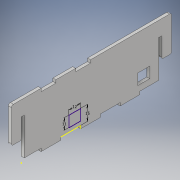
# Autodesk Inventor part: side_v2
Saved by Autodesk Inventor 2017.2 (Build 212233000, 233)
## iProperties
Created: 2017-06-09
Part Number: side_v2
Material: Generic
Document SubType Name: Modeling
Designer: SandeepSH
Density: 1 g/cm^3
Appearance: Default
Author: SandeepSH
Autodesk Inventor part; units mm, degrees
ref_plane "YZ Plane" through (0, 0, 0) normal (1, 0, 0) x (0, 1, 0)
ref_plane "XZ Plane" through (0, 0, 0) normal (0, 1, 0) x (-1, 0, 0)
ref_plane "XY Plane" through (0, 0, 0) normal (0, 0, 1) x (1, 0, 0)
sketch "Sketch1" plane through (0, 0, 0) normal (1, 0, 0) x (0, 1, 0)
  line L0 (0, 0) -> (55.5, 0)
  line L1 (55.5, 0) -> (55.5, -142)
  line L2 (55.5, -142) -> (0, -142)
  line L3 (0, -142) -> (0, 0)
  dimension "d0" = 55.5
  dimension "d1" = 142
  constraints: 8 end point, 2 parallel, 1 horizontal, 1 perpendicular
  measures "d0" distance of L1.end L2.end
  measures "d1" distance of L0.end L1.end
extrude "Extrusion1" add sketch "Sketch1" along normal blind 3
sketch "Sketch2" plane through (3, 0, 0) normal (1, 0, 0) x (0, 0, -1)
  line L0 (0, 0) -> (142, 0) projected
  line L1 (0, 0) -> (20, 0)
  line L2 (20, 0) -> (20, 3)
  line L3 (20, 3) -> (0, 3)
  line L4 (0, 3) -> (0, 0)
  line L5 (40, 0) -> (60, 0)
  line L6 (60, 0) -> (60, 3)
  line L7 (60, 3) -> (40, 3)
  line L8 (40, 3) -> (40, 0)
  line L9 (80, 0) -> (100, 0)
  line L10 (100, 0) -> (100, 3)
  line L11 (100, 3) -> (80, 3)
  line L12 (80, 3) -> (80, 0)
  line L13 (142, 0) -> (120, 0)
  line L14 (120, 0) -> (120, 3)
  line L15 (120, 3) -> (142, 3)
  line L16 (142, 3) -> (142, 0)
  line L17 (142, 55.5) -> (0, 55.5) projected
  line L18 (20, 55.5) -> (35, 55.5)
  line L19 (35, 55.5) -> (35, 52.5)
  line L20 (35, 52.5) -> (20, 52.5)
  line L21 (20, 52.5) -> (20, 55.5)
  line L22 (0, 55.5) -> (0, 0) projected
  line L23 (55, 55.5) -> (70, 55.5)
  line L24 (70, 55.5) -> (70, 52.5)
  line L25 (70, 52.5) -> (55, 52.5)
  line L26 (55, 52.5) -> (55, 55.5)
  line L27 (0, 3) -> (3, 3)
  line L28 (3, 3) -> (3, 40.5)
  line L29 (3, 40.5) -> (0, 40.5)
  line L30 (0, 40.5) -> (0, 3)
  line L31 (142, 3) -> (139, 3)
  line L32 (139, 3) -> (139, 40.5)
  line L33 (139, 40.5) -> (142, 40.5)
  line L34 (142, 40.5) -> (142, 3)
  dimension "d4" = 20
  dimension "d5" = 3
  dimension "d6" = 20
  dimension "d7" = 20
  dimension "d8" = 3
  dimension "d9" = 20
  dimension "d10" = 20
  dimension "d11" = 3
  dimension "d12" = 20
  dimension "d13" = 15
  dimension "d14" = 3
  dimension "d17" = 20
  dimension "d18" = 15
  dimension "d19" = 20
  dimension "d20" = 3
  dimension "d21" = 15
  dimension "d22" = 3
  dimension "d23" = 15
  constraints: 64 end point, 16 parallel, 8 horizontal, 8 perpendicular, 5 point on line
  measures "d4" distance of L3.end L2.end
  measures "d5" distance of L2.end L1.end
  measures "d6" distance of L7.end L6.end
  measures "d7" distance of L11.end L10.end
  measures "d8" distance of L10.end L9.end
  measures "d9" distance between parallel lines of L8 L2
  measures "d10" distance between parallel lines of L12 L6
  measures "d11" distance of L13.end L14.end
  measures "d12" distance between parallel lines of L14 L10
  measures "d13" distance of L19.end L20.end
  measures "d14" distance of L18.end L19.end
  measures "d17" distance between parallel lines of L21 L22
  measures "d18" distance of L24.end L25.end
  measures "d19" distance between parallel lines of L26 L19
  measures "d20" distance of L29.end L28.end
  measures "d21" distance between parallel lines of L17 L29
  measures "d22" distance of L32.end L33.end
  measures "d23" distance between parallel lines of L17 L33
extrude "Extrusion2" cut sketch "Sketch2" against normal through all
sketch "Sketch3" plane through (3, 0, 0) normal (1, 0, 0) x (0, 0, -1)
  line L0 (74, 26.1259) -> (74, 15.3243)
  line L1 (0, 55.5) -> (0, 40.5) projected
  line L2 (0, 55.5) -> (-10, 55.5)
  line L3 (-10, 55.5) -> (-10, 20)
  line L4 (-10, 20) -> (0, 20)
  line L5 (0, 20) -> (0, 55.5)
  line L6 (20, 0) -> (40, 0) projected
  line L7 (139, 3) -> (139, 40.5) projected
  line L8 (142, 55.5) -> (142, 40.5) projected
  line L9 (142, 55.5) -> (152, 55.5)
  line L10 (152, 55.5) -> (152, 20)
  line L11 (152, 20) -> (142, 20)
  line L12 (142, 20) -> (142, 55.5)
  line L13 (100, 0) -> (120, 0) projected
  point P0 (0, 0)
  dimension "d26" = 10
  dimension "d27" = 20
  dimension "d28" = 65
  dimension "d29" = 10
  dimension "d30" = 20
  constraints: 18 end point, 4 parallel, 2 horizontal, 2 perpendicular, 1 vertical
  measures "d26" distance of L4.end L3.end
  measures "d27" distance between parallel lines of L6 L4
  measures "d28" distance between parallel lines of L7 L0
  measures "d29" distance of L10.end L11.end
  measures "d30" distance between parallel lines of L13 L11
extrude "Extrusion3" add sketch "Sketch3" against normal blind 3
fillet "Fillet1" radius 2 6 edges at (1.5, 55.5, 10) (1.5, 20, 10) (1.5, 20, -142) (1.5, 55.5, -152) (1.5, 20, -152) (1.5, 20, 0) curvature continuous yes
sketch "Sketch4" plane through (3, 0, 0) normal (1, 0, 0) x (0, 0, -1)
  line L0 (60, 7) -> (48, 7)
  line L1 (48, 7) -> (48, 18)
  line L2 (48, 18) -> (60, 18)
  line L3 (60, 18) -> (60, 7)
  line L4 (60, 3) -> (60, 0) projected
  line L5 (40, 3) -> (60, 3) projected
  point P0 (0, 0)
  dimension "d34" = 12
  dimension "d35" = 11
  dimension "d36" = 15
  constraints: 8 end point, 2 parallel, 1 collinear, 1 horizontal, 1 perpendicular
  measures "d34" distance of L1.end L2.end
  measures "d35" distance of L0.end L1.end
  measures "d36" distance between parallel lines of L5 L2
sketch "Sketch5" plane through (3, 0, 0) normal (1, 0, 0) x (0, 0, -1)
  line L0 (118, 9) -> (130, 9)
  line L1 (130, 9) -> (130, 20)
  line L2 (130, 20) -> (118, 20)
  line L3 (118, 20) -> (118, 9)
  line L4 (80, 3) -> (100, 3) projected
  line L5 (139, 3) -> (139, 40.5) projected
  point P0 (0, 0)
  dimension "d39" = 12
  dimension "d40" = 11
  dimension "d41" = 17
  dimension "d44" = 9
  constraints: 8 end point, 2 parallel, 1 horizontal, 1 perpendicular
  measures "d39" distance of L2.end L1.end
  measures "d40" distance of L1.end L0.end
  measures "d41" distance between parallel lines of L4 L2
  measures "d44" distance between parallel lines of L5 L1
extrude "Extrusion5" cut sketch "Sketch5" against normal through all
equation "\"d9\" = d4"
equation "\"d10\" = d6"
equation "\"d12\" = d7"
body "Solid1"
